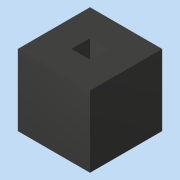
# Autodesk Inventor part: PinBlock
Saved by Autodesk Inventor 2017 (Build 210142000, 142)
## iProperties
Created: 2017-01-25
Part Number: PinBlock
Material: ABS Plastic
Document SubType Name: Modeling
Designer: techn
Density: 1.06 g/cm^3
Appearance: Smooth - Black
Author: techn
Autodesk Inventor part; units mm, degrees
ref_plane "YZ Plane" through (0, 0, 0) normal (1, 0, 0) x (0, 1, 0)
ref_plane "XZ Plane" through (0, 0, 0) normal (0, 1, 0) x (-1, 0, 0)
ref_plane "XY Plane" through (0, 0, 0) normal (0, 0, 1) x (1, 0, 0)
sketch "Sketch2" plane through (0, 0, 0) normal (0, 1, 0) x (-1, 0, 0)
  line L0 (0, 0) -> (2.54, 0)
  line L1 (2.54, 0) -> (2.54, -2.54)
  line L2 (2.54, -2.54) -> (0, -2.54)
  line L3 (0, -2.54) -> (0, 0)
  dimension "d0" = 2.54
  dimension "d1" = 2.54
  constraints: 8 end point, 2 parallel, 1 horizontal, 1 perpendicular
  measures "d0" distance of L1.end L2.end
  measures "d1" distance of L0.end L1.end
extrude "Extrusion1" add sketch "Sketch2" along normal blind 2.5
sketch "Sketch3" plane through (0, 2.5, 0) normal (0, 1, 0) x (1, 0, 0)
  line L0 (-2.54, 0) -> (0, 0) projected
  line L1 (0, 0) -> (0, 2.54) projected
  line L2 (0, 2.54) -> (-2.54, 2.54) projected
  line L3 (-2.54, 2.54) -> (-2.54, 0) projected
  line L4 (-0.945, 1.595) -> (-1.595, 1.595)
  line L5 (-1.595, 1.595) -> (-1.595, 0.945)
  line L6 (-1.595, 0.945) -> (-0.945, 0.945)
  line L7 (-0.945, 0.945) -> (-0.945, 1.595)
  dimension "d4" = 0.65
  dimension "d5" = 0.65
  dimension "d6" = 0.945
  dimension "d7" = 0.945
  constraints: 8 end point, 2 parallel, 1 horizontal, 1 perpendicular
  measures "d4" distance of L6.end L5.end
  measures "d5" distance of L5.end L4.end
  measures "d6" distance between parallel lines of L0 L6
  measures "d7" distance between parallel lines of L3 L5
extrude "Extrusion2" cut sketch "Sketch3" against normal blind 2.5 contours L7 L6 L5 L4
equation "\"d7\" = d6"
body "Solid1"
